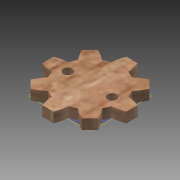
# Autodesk Inventor part: tandwiel(ja)
Saved by Autodesk Inventor 2015 (Build 190159000, 159)
## iProperties
Created: 2016-01-31
Part Number: tandwiel(ja)
Material: Generic
Document SubType Name: Modeling
Designer: david
Density: 1 g/cm^3
Appearance: Birch - Natural Polished
Mass: 1.9265 g
Surface Area: 15.9465 cm^2
Volume: 1.9265 cm^3
Author: david
Autodesk Inventor part; units mm, degrees
ref_plane "YZ Plane" through (0, 0, 0) normal (1, 0, 0) x (0, 1, 0)
ref_plane "XZ Plane" through (0, 0, 0) normal (0, 1, 0) x (-1, 0, 0)
ref_plane "XY Plane" through (0, 0, 0) normal (0, 0, 1) x (1, 0, 0)
ref_plane "Work Plane1" through (0, 0, 0) normal (0, 0, -1) x (-1, 0, 0)
sketch "Sketch3" plane through (0, 0, 0) normal (0, 0, -1) x (-1, 0, 0)
  circle A0 centre (0, 0) radius 11
  line L0 (-15.4, 0) -> (15.4, 0) projected
  dimension "d19" = 22
  constraints: 1 centre point, 1 coincident
  measures "d19" diameter of A0
extrude "Extrusion3" add sketch "Sketch3" against normal blind 3.6
sketch "Sketch4" plane through (0, 0, 3.6) normal (0, 0, 1) x (1, 0, 0)
  arc A0 (10.583, -3) -> (10.583, 3) centre (0, 0) ccw
  line L0 (-16.2075, 0) -> (20.2449, 0) projected
  line L1 (15, 0) -> (15, 2)
  arc A1 (15, 2) -> (10.583, 3) centre (9.5173, -11.9621) ccw
  line L2 (15, 0) -> (15, -2)
  arc A2 (10.583, -3) -> (15, -2) centre (9.5173, 11.9621) ccw
  dimension "d22" = 2
  dimension "d23" = 3
  dimension "d24" = 15
  dimension "d25" = 15
  dimension "d35" = 11
  constraints: 6 point on circle, 4 end point, 3 centre point, 3 symmetric about line, 1 coincident, 1 point on line, 1 vertical, 1 other
  measures "d22" distance of L1.start L1.end
  measures "d23" distance from line of L0 A0.end
  measures "d24" radius of A1
  measures "d25" distance from line of point (0, 0) L1
  measures "d35" radius of A0
extrude "Extrusion4" add sketch "Sketch4" against normal blind 3.6
sketch "Sketch2" plane through (0, 0, 0) normal (0, 0, -1) x (-1, 0, 0)
  line L0 (-9.8, -2.6) -> (-6, -2.6)
  line L1 (-6, -2.6) -> (-6, 2.6)
  line L2 (-6, 2.6) -> (-9.8, 2.6)
  line L3 (-9.8, 2.6) -> (-9.8, -2.6)
  line L4 (-9.8, -2.6) -> (-6, 2.6) construction
  line L5 (-6, -2.6) -> (-9.8, 2.6) construction
  line L6 (0, -27.5637) -> (0, 32.5752)
  line L7 (9.8, -2.6) -> (6, -2.6)
  line L8 (6, -2.6) -> (6, 2.6)
  line L9 (6, 2.6) -> (9.8, 2.6)
  line L10 (9.8, 2.6) -> (9.8, -2.6)
  line L11 (9.8, -2.6) -> (6, 2.6) construction
  line L12 (6, -2.6) -> (9.8, 2.6) construction
  circle A0 centre (-7.9, 0) radius 1.625
  circle A1 centre (7.9, 0) radius 1.625
  point P0 (0, 0)
  dimension "d31" = 6
  dimension "d32" = 0
  dimension "d33" = 3.25
  dimension "d34" = 3.25
  constraints: 26 end point, 5 symmetric about line, 4 midpoint, 2 centre point, 2 coincident, 2 parallel, 1 horizontal, 1 perpendicular, 1 vertical
  measures "d31" distance from line of point (0, 0) L1
  measures "d32" distance from line of point (0, 0) L6
  measures "d33" diameter of A0
  measures "d34" diameter of A1
extrude "Extrusion2" cut sketch "Sketch2" against normal blind 3.6 contours A0 | A1
pattern_circular "Circular Pattern1" count 8 over 360 about axis through (0, 0, 0) along (0, 0, 1) of "Extrusion4"
body "Solid1"
